Autodesk Fusion 360 part; units mm, degrees
note: some values were not read from the file. Set by a fixed rule: which sketch regions a step uses.
(part 3 of 15)
  line L1668 (302.273, -82.2438) -> (302.188, -82.0789)
  line L1669 (24.5588, -81.825) -> (24.4325, -81.5723)
  line L1670 (32.1614, -81.3271) -> (32.215, -81.5045)
  line L1671 (302.388, -82.3891) -> (302.273, -82.2438)
  line L1672 (302.137, -81.9006) -> (302.122, -81.7159)
  line L1673 (302.198, -81.3549) -> (302.288, -81.1924)
  line L1674 (303.95, -81.3671) -> (304.003, -81.5446)
  line L1675 (303.052, -82.6789) -> (302.867, -82.657)
  line L1676 (303.236, -82.6647) -> (303.052, -82.6789)
  line L1677 (32.0744, -81.1633) -> (32.1614, -81.3271)
  line L1678 (31.4741, -80.7585) -> (31.6512, -80.8133)
  line L1679 (302.188, -82.0789) -> (302.137, -81.9006)
  line L1680 (302.142, -81.5316) -> (302.198, -81.3549)
  line L1681 (302.407, -81.0504) -> (302.551, -80.9342)
  line L1682 (302.716, -80.8483) -> (302.893, -80.796)
  line L1683 (31.6512, -80.8133) -> (31.8143, -80.9015)
  line L1684 (31.8143, -80.9015) -> (31.9572, -81.0197)
  line L1685 (24.801, -79.4609) -> (25.0054, -79.2659)
  line L1686 (25.2353, -79.1017) -> (25.486, -78.9714)
  line L1687 (303.746, -81.0597) -> (303.863, -81.2034)
  line L1688 (24.2812, -80.7441) -> (24.31, -80.4631)
  line L1689 (304.003, -81.5446) -> (304.021, -81.7291)
  line L1690 (303.262, -80.7985) -> (303.44, -80.8534)
  line L1691 (85.9153, -105.918) -> (85.7941, -106.059)
  line L1692 (84.7587, -106.241) -> (84.5968, -106.151)
  line L1693 (274.699, -101.972) -> (274.897, -102.173)
  line L1694 (84.5968, -106.151) -> (84.4556, -106.031)
  line L1695 (-66.507, -105.451) -> (-66.5655, -105.627)
  line L1696 (-68.3832, -105.227) -> (-68.3626, -105.043)
  line L1697 (274.897, -102.173) -> (275.065, -102.4)
  line L1698 (85.1191, -106.321) -> (84.935, -106.299)
  line L1699 (84.3404, -105.885) -> (84.2557, -105.721)
  line L1700 (84.2097, -105.173) -> (84.2658, -104.997)
  line L1701 (-66.7782, -105.929) -> (-66.9243, -106.043)
  line L1702 (-67.2684, -106.176) -> (-67.4532, -106.19)
  line L1703 (84.1891, -105.358) -> (84.2097, -105.173)
  line L1704 (-66.9243, -106.043) -> (-67.0898, -106.126)
  line L1705 (85.1456, -104.421) -> (85.33, -104.44)
  line L1706 (84.2658, -104.997) -> (84.3551, -104.834)
  line L1707 (-67.0652, -104.365) -> (-66.9021, -104.453)
  line L1708 (-67.4532, -106.19) -> (-67.6373, -106.168)
  line L1709 (-68.3677, -105.412) -> (-68.3832, -105.227)
  line L1710 (-67.4267, -104.291) -> (-67.2423, -104.31)
  line L1711 (-68.098, -104.562) -> (-67.9535, -104.446)
  line L1712 (273.689, -101.497) -> (273.964, -101.56)
  line L1713 (84.935, -106.299) -> (84.7587, -106.241)
  line L1714 (84.4556, -106.031) -> (84.3404, -105.885)
  line L1715 (274.474, -101.8) -> (274.699, -101.972)
  line L1716 (-68.3166, -105.59) -> (-68.3677, -105.412)
  line L1717 (273.964, -101.56) -> (274.227, -101.662)
  line L1718 (-68.3626, -105.043) -> (-68.3065, -104.866)
  line L1719 (-67.6114, -104.307) -> (-67.4267, -104.291)
  line L1720 (-68.3065, -104.866) -> (-68.2172, -104.704)
  line L1721 (274.227, -101.662) -> (274.474, -101.8)
  line L1722 (275.065, -102.4) -> (275.199, -102.649)
  line L1723 (86.0173, -105.009) -> (86.0709, -105.186)
  line L1724 (249.992, -105.959) -> (249.871, -106.099)
  line L1725 (78.199, -104.986) -> (78.1482, -104.708)
  line L1726 (78.4147, -105.507) -> (78.2884, -105.254)
  line L1727 (85.9303, -104.845) -> (86.0173, -105.009)
  line L1728 (248.432, -104.874) -> (248.551, -104.732)
  line L1729 (86.089, -105.371) -> (86.0886, -105.397)
  line L1730 (249.38, -106.346) -> (249.196, -106.361)
  line L1731 (78.6569, -103.143) -> (78.8613, -102.948)
  line L1732 (248.551, -104.732) -> (248.695, -104.616)
  line L1733 (78.2884, -105.254) -> (78.199, -104.986)
  line L1734 (250.166, -105.411) -> (250.165, -105.437)
  line L1735 (250.165, -105.437) -> (250.142, -105.621)
  line L1736 (79.2282, -106.271) -> (78.9861, -106.125)
  line L1737 (78.234, -103.871) -> (78.3401, -103.609)
  line L1738 (250.007, -104.885) -> (250.094, -105.049)
  line L1739 (248.532, -106.071) -> (248.417, -105.926)
  line L1740 (249.012, -106.339) -> (248.835, -106.281)
  line L1741 (85.6702, -104.583) -> (85.8131, -104.701)
  line L1742 (248.286, -105.213) -> (248.342, -105.037)
  line L1743 (86.0709, -105.186) -> (86.089, -105.371)
  line L1744 (86.0886, -105.397) -> (86.0654, -105.581)
  line L1745 (249.559, -106.297) -> (249.38, -106.346)
  line L1746 (85.5071, -104.495) -> (85.6702, -104.583)
  line L1747 (250.147, -105.226) -> (250.166, -105.411)
  line L1748 (78.8613, -102.948) -> (79.0912, -102.783)
  line L1749 (78.1482, -104.708) -> (78.1371, -104.426)
  line L1750 (79.0912, -102.783) -> (79.3419, -102.653)
  line L1751 (78.1371, -104.426) -> (78.1659, -104.145)
  line L1752 (249.196, -106.361) -> (249.012, -106.339)
  line L1753 (85.33, -104.44) -> (85.5071, -104.495)
  line L1754 (248.332, -105.761) -> (248.281, -105.582)
  line L1755 (250.142, -105.621) -> (250.083, -105.797)
  line L1756 (249.222, -104.461) -> (249.407, -104.48)
  line L1757 (248.673, -106.191) -> (248.532, -106.071)
  line L1758 (249.725, -106.213) -> (249.559, -106.297)
  line L1759 (85.8131, -104.701) -> (85.9303, -104.845)
  line L1760 (249.871, -106.099) -> (249.725, -106.213)
  line L1761 (248.835, -106.281) -> (248.673, -106.191)
  line L1762 (248.342, -105.037) -> (248.432, -104.874)
  line L1763 (86.0069, -105.757) -> (85.9153, -105.918)
  line L1764 (248.417, -105.926) -> (248.332, -105.761)
  line L1765 (248.266, -105.398) -> (248.286, -105.213)
  line L1766 (248.281, -105.582) -> (248.266, -105.398)
  line L1767 (250.083, -105.797) -> (249.992, -105.959)
  line L1768 (248.695, -104.616) -> (248.86, -104.53)
  line L1769 (248.86, -104.53) -> (249.038, -104.478)
  line L1770 (249.038, -104.478) -> (249.222, -104.461)
  line L1771 (84.961, -104.438) -> (85.1456, -104.421)
  line L1772 (-67.2423, -104.31) -> (-67.0652, -104.365)
  line L1773 (84.2046, -105.542) -> (84.1891, -105.358)
  line L1774 (84.6188, -104.576) -> (84.7831, -104.49)
  line L1775 (85.304, -106.306) -> (85.1191, -106.321)
  line L1776 (85.7941, -106.059) -> (85.648, -106.173)
  line L1777 (84.7831, -104.49) -> (84.961, -104.438)
  line L1778 (84.4743, -104.692) -> (84.6188, -104.576)
  line L1779 (84.3551, -104.834) -> (84.4743, -104.692)
  line L1780 (-66.7592, -104.571) -> (-66.6421, -104.715)
  line L1781 (-66.6421, -104.715) -> (-66.555, -104.879)
  line L1782 (-66.555, -104.879) -> (-66.5014, -105.056)
  line L1783 (86.0654, -105.581) -> (86.0069, -105.757)
  line L1784 (-66.9021, -104.453) -> (-66.7592, -104.571)
  line L1785 (84.2557, -105.721) -> (84.2046, -105.542)
  line L1786 (-66.4833, -105.241) -> (-66.4837, -105.267)
  line L1787 (-66.5014, -105.056) -> (-66.4833, -105.241)
  line L1788 (85.4825, -106.257) -> (85.304, -106.306)
  line L1789 (85.648, -106.173) -> (85.4825, -106.257)
  line L1790 (227.735, -91.279) -> (227.912, -91.3338)
  line L1791 (100.763, -89.5821) -> (101.013, -89.4519)
  line L1792 (228.494, -92.2361) -> (228.47, -92.42)
  line L1793 (228.412, -92.596) -> (228.32, -92.7572)
  line L1794 (100.086, -92.3055) -> (99.96, -92.0527)
  line L1795 (228.32, -92.7572) -> (228.199, -92.8975)
  line L1796 (228.335, -91.6839) -> (228.422, -91.8476)
  line L1797 (228.053, -93.0117) -> (227.887, -93.0953)
  line L1798 (227.887, -93.0953) -> (227.709, -93.1451)
  line L1799 (107.466, -92.8575) -> (107.32, -92.9716)
  line L1800 (107.342, -91.3819) -> (107.485, -91.5001)
  line L1801 (226.745, -92.7242) -> (226.661, -92.5593)
  line L1802 (227.912, -91.3338) -> (228.075, -91.422)
  line L1803 (101.557, -89.3031) -> (101.839, -89.2876)
  line L1804 (226.671, -91.8353) -> (226.76, -91.6729)
  line L1805 (107.678, -92.5559) -> (107.587, -92.7171)
  line L1806 (107.32, -92.9716) -> (107.154, -93.0552)
  line L1807 (107.179, -91.2937) -> (107.342, -91.3819)
  line L1808 (227.34, -93.1374) -> (227.164, -93.0801)
  line L1809 (227.164, -93.0801) -> (227.002, -92.9897)
  line L1810 (226.594, -92.1963) -> (226.615, -92.0121)
  line L1811 (226.615, -92.0121) -> (226.671, -91.8353)
  line L1812 (107.485, -91.5001) -> (107.602, -91.6438)
  line L1813 (107.154, -93.0552) -> (106.976, -93.1051)
  line L1814 (227.551, -91.2596) -> (227.735, -91.279)
  line L1815 (107.602, -91.6438) -> (107.689, -91.8075)
  line L1816 (227.524, -93.1594) -> (227.34, -93.1374)
  line L1817 (226.61, -92.3811) -> (226.594, -92.1963)
  line L1818 (107.743, -91.985) -> (107.761, -92.1695)
  line L1819 (226.861, -92.8695) -> (226.745, -92.7242)
  line L1820 (107.689, -91.8075) -> (107.743, -91.985)
  line L1821 (227.366, -91.2764) -> (227.551, -91.2596)
  line L1822 (107.587, -92.7171) -> (107.466, -92.8575)
  line L1823 (226.76, -91.6729) -> (226.879, -91.5308)
  line L1824 (227.188, -91.3287) -> (227.366, -91.2764)
  line L1825 (226.661, -92.5593) -> (226.61, -92.3811)
  line L1826 (107.002, -91.2389) -> (107.179, -91.2937)
  line L1827 (-17.1187, -94.0653) -> (-16.9544, -93.9794)
  line L1828 (-26.4131, -92.1654) -> (-26.236, -92.2202)
  line L1829 (-25.8129, -92.5702) -> (-25.7258, -92.7339)
  line L1830 (-27.5386, -93.2674) -> (-27.5541, -93.0827)
  line L1831 (-26.236, -92.2202) -> (-26.0729, -92.3084)
  line L1832 (-17.3824, -94.3235) -> (-17.2632, -94.1815)
  line L1833 (-17.4717, -94.486) -> (-17.3824, -94.3235)
  line L1834 (-25.6723, -92.9114) -> (-25.6542, -93.096)
  line L1835 (233.398, -89.5178) -> (233.645, -89.6558)
  line L1836 (-16.4336, -95.7958) -> (-16.6184, -95.81)
  line L1837 (-25.6778, -93.3064) -> (-25.7363, -93.4824)
  line L1838 (-17.3971, -95.3748) -> (-17.4818, -95.2099)
  line L1839 (-25.6545, -93.1225) -> (-25.6778, -93.3064)
  line L1840 (-16.9544, -93.9794) -> (-16.7765, -93.927)
  line L1841 (-26.7822, -92.1628) -> (-26.5975, -92.146)
  line L1842 (-27.5541, -93.0827) -> (-27.5334, -92.8984)
  line L1843 (-27.2688, -92.4172) -> (-27.1244, -92.301)
  line L1844 (-26.4392, -94.0315) -> (-26.6241, -94.0457)
  line L1845 (233.645, -89.6558) -> (233.869, -89.8272)
  line L1846 (232.86, -89.3521) -> (233.135, -89.4159)
  line L1847 (-26.8082, -94.0238) -> (-26.9845, -93.9665)
  line L1848 (-16.255, -95.7459) -> (-16.4336, -95.7958)
  line L1849 (-16.5919, -93.9102) -> (-16.4075, -93.9296)
  line L1850 (-16.6184, -95.81) -> (-16.8025, -95.7881)
  line L1851 (233.135, -89.4159) -> (233.398, -89.5178)
  line L1852 (-16.8025, -95.7881) -> (-16.9789, -95.7308)
  line L1853 (-17.5484, -94.847) -> (-17.5278, -94.6627)
  line L1854 (-25.9301, -92.4266) -> (-25.8129, -92.5702)
  line L1855 (-16.9789, -95.7308) -> (-17.1407, -95.6403)
  line L1856 (-16.7765, -93.927) -> (-16.5919, -93.9102)
  line L1857 (-25.6542, -93.096) -> (-25.6545, -93.1225)
  line L1858 (-25.7363, -93.4824) -> (-25.8279, -93.6436)
  line L1859 (233.869, -89.8272) -> (234.068, -90.0285)
  line L1860 (-27.2875, -93.7559) -> (-27.4027, -93.6106)
  line L1861 (-27.4773, -92.7217) -> (-27.388, -92.5592)
  line L1862 (-26.96, -92.2151) -> (-26.7822, -92.1628)
  line L1863 (234.068, -90.0285) -> (234.235, -90.2558)
  line L1864 (234.235, -90.2558) -> (234.37, -90.5044)
  line L1865 (234.37, -90.5044) -> (234.467, -90.7695)
  line L1866 (234.467, -90.7695) -> (234.527, -91.0456)
  line L1867 (234.527, -91.0456) -> (234.547, -91.3274)
  line L1868 (-26.0951, -93.8981) -> (-26.2606, -93.9817)
  line L1869 (-25.949, -93.7839) -> (-26.0951, -93.8981)
  line L1870 (-27.388, -92.5592) -> (-27.2688, -92.4172)
  line L1871 (-27.1463, -93.876) -> (-27.2875, -93.7559)
  line L1872 (-27.4875, -93.4457) -> (-27.5386, -93.2674)
  line L1873 (-27.1244, -92.301) -> (-26.96, -92.2151)
  line L1874 (-25.8279, -93.6436) -> (-25.949, -93.7839)
  line L1875 (231.752, -89.4919) -> (232.019, -89.3983)
  line L1876 (230.61, -91.8248) -> (230.559, -91.5469)
  line L1877 (230.893, -90.2033) -> (231.067, -89.9814)
  line L1878 (233.773, -92.9078) -> (233.538, -93.0647)
  line L1879 (231.178, -92.7854) -> (230.986, -92.5779)
  line L1880 (234.165, -92.503) -> (233.983, -92.7193)
  line L1881 (234.428, -92.0049) -> (234.314, -92.2633)
  line L1882 (-26.5975, -92.146) -> (-26.4131, -92.1654)
  line L1883 (-26.2606, -93.9817) -> (-26.4392, -94.0315)
  line L1884 (230.576, -90.9836) -> (230.645, -90.7094)
  line L1885 (-26.6241, -94.0457) -> (-26.8082, -94.0238)
  line L1886 (-26.9845, -93.9665) -> (-27.1463, -93.876)
  line L1887 (-27.5334, -92.8984) -> (-27.4773, -92.7217)
  line L1888 (234.314, -92.2633) -> (234.165, -92.503)
  line L1889 (230.699, -92.0928) -> (230.61, -91.8248)
  line L1890 (234.547, -91.3274) -> (234.543, -91.453)
  line L1891 (233.283, -93.187) -> (233.014, -93.2722)
  line L1892 (233.983, -92.7193) -> (233.773, -92.9078)
  line L1893 (231.397, -92.9637) -> (231.178, -92.7854)
  line L1894 (231.272, -89.7864) -> (231.502, -89.6222)
  line L1895 (233.538, -93.0647) -> (233.283, -93.187)
  line L1896 (231.502, -89.6222) -> (231.752, -89.4919)
  line L1897 (234.543, -91.453) -> (234.505, -91.733)
  line L1898 (-27.4027, -93.6106) -> (-27.4875, -93.4457)
  line L1899 (230.645, -90.7094) -> (230.751, -90.4476)
  line L1900 (230.825, -92.3455) -> (230.699, -92.0928)
  line L1901 (234.505, -91.733) -> (234.428, -92.0049)
  line L1902 (230.548, -91.2646) -> (230.576, -90.9836)
  line L1903 (232.172, -93.292) -> (231.899, -93.2196)
  line L1904 (230.751, -90.4476) -> (230.893, -90.2033)
  line L1905 (231.067, -89.9814) -> (231.272, -89.7864)
  line L1906 (232.453, -93.3252) -> (232.172, -93.292)
  line L1907 (230.986, -92.5779) -> (230.825, -92.3455)
  line L1908 (231.899, -93.2196) -> (231.639, -93.1095)
  line L1909 (230.559, -91.5469) -> (230.548, -91.2646)
  line L1910 (103.426, -92.4629) -> (103.244, -92.6792)
  line L1911 (233.014, -93.2722) -> (232.735, -93.3186)
  line L1912 (232.735, -93.3186) -> (232.453, -93.3252)
  line L1913 (103.804, -91.413) -> (103.766, -91.6929)
  line L1914 (101.433, -93.2519) -> (101.16, -93.1795)
  line L1915 (102.906, -89.6158) -> (103.13, -89.7872)
  line L1916 (102.659, -89.4777) -> (102.906, -89.6158)
  line L1917 (103.496, -90.2157) -> (103.631, -90.4643)
  line L1918 (103.034, -92.8677) -> (102.799, -93.0246)
  line L1919 (102.275, -93.2321) -> (101.996, -93.2785)
  line L1920 (103.631, -90.4643) -> (103.728, -90.7294)
  line L1921 (103.766, -91.6929) -> (103.69, -91.9649)
  line L1922 (100.247, -92.5379) -> (100.086, -92.3055)
  line L1923 (231.639, -93.1095) -> (231.397, -92.9637)
  line L1924 (102.799, -93.0246) -> (102.544, -93.1469)
  line L1925 (101.996, -93.2785) -> (101.714, -93.2852)
  line L1926 (232.296, -89.3432) -> (232.578, -89.3277)
  line L1927 (100.9, -93.0694) -> (100.658, -92.9237)
  line L1928 (100.658, -92.9237) -> (100.439, -92.7453)
  line L1929 (100.439, -92.7453) -> (100.247, -92.5379)
  line L1930 (103.329, -89.9885) -> (103.496, -90.2157)
  line L1931 (102.121, -89.312) -> (102.396, -89.3758)
  line L1932 (103.788, -91.0056) -> (103.808, -91.2874)
  line L1933 (103.13, -89.7872) -> (103.329, -89.9885)
  line L1934 (102.396, -89.3758) -> (102.659, -89.4777)
  line L1935 (103.808, -91.2874) -> (103.804, -91.413)
  line L1936 (101.714, -93.2852) -> (101.433, -93.2519)
  line L1937 (102.544, -93.1469) -> (102.275, -93.2321)
  line L1938 (227.709, -93.1451) -> (227.524, -93.1594)
  line L1939 (99.8706, -91.7848) -> (99.8199, -91.5068)
  line L1940 (100.154, -90.1632) -> (100.329, -89.9413)
  line L1941 (99.8088, -91.2246) -> (99.8376, -90.9435)
  line L1942 (100.329, -89.9413) -> (100.533, -89.7463)
  line L1943 (99.9057, -90.6693) -> (100.012, -90.4075)
  line L1944 (228.218, -91.5402) -> (228.335, -91.6839)
  line L1945 (100.533, -89.7463) -> (100.763, -89.5821)
  line L1946 (228.075, -91.422) -> (228.218, -91.5402)
  line L1947 (103.575, -92.2232) -> (103.426, -92.4629)
  line L1948 (228.422, -91.8476) -> (228.476, -92.0251)
  line L1949 (99.8199, -91.5068) -> (99.8088, -91.2246)
  line L1950 (228.476, -92.0251) -> (228.494, -92.2096)
  line L1951 (99.8376, -90.9435) -> (99.9057, -90.6693)
  line L1952 (228.494, -92.2096) -> (228.494, -92.2361)
  line L1953 (101.16, -93.1795) -> (100.9, -93.0694)
  line L1954 (103.728, -90.7294) -> (103.788, -91.0056)
  line L1955 (232.019, -89.3983) -> (232.296, -89.3432)
  line L1956 (103.244, -92.6792) -> (103.034, -92.8677)
  line L1957 (232.578, -89.3277) -> (232.86, -89.3521)
  line L1958 (103.69, -91.9649) -> (103.575, -92.2232)
  line L1959 (99.96, -92.0527) -> (99.8706, -91.7848)
  line L1960 (100.012, -90.4075) -> (100.154, -90.1632)
  line L1961 (101.28, -89.3583) -> (101.557, -89.3031)
  line L1962 (101.013, -89.4519) -> (101.28, -89.3583)
  line L1963 (228.199, -92.8975) -> (228.053, -93.0117)
  line L1964 (228.47, -92.42) -> (228.412, -92.596)
  line L1965 (101.839, -89.2876) -> (102.121, -89.312)
  line L1966 (288.551, -103.613) -> (288.569, -103.798)
  line L1967 (287.599, -104.748) -> (287.415, -104.726)
  line L1968 (47.614, -103.396) -> (47.6676, -103.573)
  line L1969 (287.238, -104.668) -> (287.077, -104.578)
  line L1970 (288.128, -104.6) -> (287.962, -104.683)
  line L1971 (286.935, -104.458) -> (286.82, -104.312)
  line L1972 (287.784, -104.733) -> (287.599, -104.748)
  line L1973 (287.263, -102.917) -> (287.441, -102.865)
  line L1974 (287.077, -104.578) -> (286.935, -104.458)
  line L1975 (47.3908, -104.446) -> (47.2447, -104.56)
  line L1976 (39.7957, -103.373) -> (39.7449, -103.095)
  line L1977 (40.2536, -101.529) -> (40.458, -101.334)
  line L1978 (288.569, -103.798) -> (288.568, -103.824)
  line L1979 (286.736, -104.147) -> (286.684, -103.969)
  line L1980 (40.458, -101.334) -> (40.6879, -101.17)
  line L1981 (286.669, -103.784) -> (286.69, -103.6)
  line L1982 (288.395, -104.345) -> (288.274, -104.486)
  line L1983 (41.7643, -100.876) -> (42.0457, -100.9)
  line L1984 (287.987, -102.922) -> (288.15, -103.01)
  line L1985 (288.274, -104.486) -> (288.128, -104.6)
  line L1986 (288.568, -103.824) -> (288.545, -104.008)
  line L1987 (40.6879, -101.17) -> (40.9386, -101.04)
  line L1988 (287.962, -104.683) -> (287.784, -104.733)
  line L1989 (288.41, -103.272) -> (288.497, -103.436)
  line L1990 (39.7626, -102.532) -> (39.8307, -102.257)
  line L1991 (47.2669, -102.97) -> (47.4098, -103.088)
  line L1992 (47.2447, -104.56) -> (47.0792, -104.643)
  line L1993 (288.545, -104.008) -> (288.487, -104.184)
  line L1994 (47.512, -104.305) -> (47.3908, -104.446)
  line L1995 (41.4822, -100.891) -> (41.7643, -100.876)
  line L1996 (286.684, -103.969) -> (286.669, -103.784)
  line L1997 (287.415, -104.726) -> (287.238, -104.668)
  line L1998 (46.9267, -102.827) -> (47.1038, -102.882)
  line L1999 (47.527, -103.232) -> (47.614, -103.396)
  line L2000 (47.6621, -103.968) -> (47.6035, -104.144)
  line L2001 (46.9006, -104.693) -> (46.7158, -104.707)
  line L2002 (47.6035, -104.144) -> (47.512, -104.305)
  line L2003 (286.746, -103.423) -> (286.835, -103.261)
  line L2004 (47.0792, -104.643) -> (46.9006, -104.693)
  line L2005 (287.099, -103.003) -> (287.263, -102.917)
  line L2006 (287.625, -102.848) -> (287.81, -102.867)
  line L2007 (286.82, -104.312) -> (286.736, -104.147)
  line L2008 (286.835, -103.261) -> (286.954, -103.119)
  line L2009 (286.69, -103.6) -> (286.746, -103.423)
  line L2010 (260.153, -103.462) -> (260.171, -103.647)
  line L2011 (47.1038, -102.882) -> (47.2669, -102.97)
  line L2012 (46.5577, -102.824) -> (46.7423, -102.808)
  line L2013 (260.099, -103.285) -> (260.153, -103.462)
  line L2014 (259.997, -104.194) -> (259.876, -104.335)
  line L2015 (47.6857, -103.758) -> (47.6853, -103.784)
  line L2016 (286.954, -103.119) -> (287.099, -103.003)
  line L2017 (287.441, -102.865) -> (287.625, -102.848)
  line L2018 (260.089, -104.033) -> (259.997, -104.194)
  line L2019 (259.876, -104.335) -> (259.73, -104.449)
  line L2020 (45.9371, -104.272) -> (45.8524, -104.107)
  line L2021 (47.6853, -103.784) -> (47.6621, -103.968)
  line L2022 (260.148, -103.857) -> (260.089, -104.033)
  line L2023 (47.4098, -103.088) -> (47.527, -103.232)
  line L2024 (45.7858, -103.744) -> (45.8064, -103.56)
  line L2025 (259.565, -104.532) -> (259.386, -104.582)
  line L2026 (46.3798, -102.877) -> (46.5577, -102.824)
  line L2027 (46.5317, -104.685) -> (46.3553, -104.628)
  line L2028 (47.6676, -103.573) -> (47.6857, -103.758)
  line L2029 (46.0523, -104.418) -> (45.9371, -104.272)
  line L2030 (46.2155, -102.963) -> (46.3798, -102.877)
  line L2031 (259.73, -104.449) -> (259.565, -104.532)
  line L2032 (46.1935, -104.538) -> (46.0523, -104.418)
  line L2033 (46.071, -103.079) -> (46.2155, -102.963)
  line L2034 (45.8013, -103.929) -> (45.7858, -103.744)
  line L2035 (45.9518, -103.221) -> (46.071, -103.079)
  line L2036 (45.8625, -103.383) -> (45.9518, -103.221)
  line L2037 (46.7423, -102.808) -> (46.9267, -102.827)
  line L2038 (259.589, -102.771) -> (259.752, -102.859)
  line L2039 (46.3553, -104.628) -> (46.1935, -104.538)
  line L2040 (259.412, -102.716) -> (259.589, -102.771)
  line L2041 (260.012, -103.121) -> (260.099, -103.285)
  line L2042 (260.171, -103.647) -> (260.171, -103.673)
  line L2043 (260.171, -103.673) -> (260.148, -103.857)
  line L2044 (259.752, -102.859) -> (259.895, -102.977)
  line L2045 (45.8524, -104.107) -> (45.8013, -103.929)
  line L2046 (45.8064, -103.56) -> (45.8625, -103.383)
  line L2047 (46.7158, -104.707) -> (46.5317, -104.685)
  line L2048 (258.338, -103.996) -> (258.287, -103.818)
  line L2049 (74.6132, -102.812) -> (74.7775, -102.726)
  line L2050 (259.017, -104.574) -> (258.841, -104.517)
  line L2051 (259.201, -104.596) -> (259.017, -104.574)
  line L2052 (258.348, -103.272) -> (258.437, -103.11)
  line L2053 (76.0117, -103.245) -> (76.0652, -103.422)
  line L2054 (258.701, -102.852) -> (258.865, -102.766)
  line L2055 (259.386, -104.582) -> (259.201, -104.596)
  line L2056 (75.9096, -104.154) -> (75.7885, -104.295)
  line L2057 (75.7885, -104.295) -> (75.6424, -104.409)
  line L2058 (258.679, -104.427) -> (258.538, -104.307)
  line L2059 (76.0833, -103.607) -> (76.083, -103.633)
  line L2060 (258.423, -104.161) -> (258.338, -103.996)
  line L2061 (75.5015, -102.731) -> (75.6646, -102.819)
  line L2062 (258.841, -104.517) -> (258.679, -104.427)
  line L2063 (76.0597, -103.817) -> (76.0012, -103.993)
  line L2064 (258.287, -103.818) -> (258.271, -103.633)
  line L2065 (258.538, -104.307) -> (258.423, -104.161)
  line L2066 (76.0652, -103.422) -> (76.0833, -103.607)
  line L2067 (76.083, -103.633) -> (76.0597, -103.817)
  line L2068 (258.271, -103.633) -> (258.292, -103.449)
  line L2069 (75.6424, -104.409) -> (75.4769, -104.492)
  line L2070 (75.14, -102.657) -> (75.3244, -102.676)
  line L2071 (278.91, -101.802) -> (279.053, -101.92)
  line L2072 (74.5912, -104.387) -> (74.45, -104.266)
  line L2073 (258.292, -103.449) -> (258.348, -103.272)
  line L2074 (76.0012, -103.993) -> (75.9096, -104.154)
  line L2075 (258.437, -103.11) -> (258.556, -102.968)
  line L2076 (259.043, -102.713) -> (259.228, -102.697)
  line L2077 (258.865, -102.766) -> (259.043, -102.713)
  line L2078 (74.3348, -104.121) -> (74.2501, -103.956)
  line L2079 (75.9246, -103.081) -> (76.0117, -103.245)
  line L2080 (75.2983, -104.542) -> (75.1134, -104.556)
  line L2081 (259.228, -102.697) -> (259.412, -102.716)
  line L2082 (75.3244, -102.676) -> (75.5015, -102.731)
  line L2083 (74.7775, -102.726) -> (74.9553, -102.673)
  line L2084 (258.556, -102.968) -> (258.701, -102.852)
  line L2085 (75.8074, -102.937) -> (75.9246, -103.081)
  line L2086 (259.895, -102.977) -> (260.012, -103.121)
  line L2087 (75.6646, -102.819) -> (75.8074, -102.937)
  line L2088 (74.9553, -102.673) -> (75.14, -102.657)
  line L2089 (75.1134, -104.556) -> (74.9293, -104.534)
  line L2090 (74.1834, -103.593) -> (74.2041, -103.409)
  line L2091 (279.311, -102.405) -> (279.329, -102.59)
  line L2092 (279.17, -102.064) -> (279.257, -102.228)
  line L2093 (295.167, -141.134) -> (295.185, -141.319)
  line L2094 (295.185, -141.319) -> (295.184, -141.345)
  line L2095 (294.578, -142.205) -> (294.4, -142.254)
  line L2096 (293.57, -140.64) -> (293.715, -140.524)
  line L2097 (293.352, -141.669) -> (293.3, -141.49)
  line L2098 (294.031, -142.247) -> (293.854, -142.189)
  line L2099 (39.2364, -141.629) -> (39.1853, -141.45)
  line L2100 (39.1853, -141.45) -> (39.1698, -141.266)
  line L2101 (40.896, -141.826) -> (40.7748, -141.967)
  line L2102 (40.2846, -142.214) -> (40.0998, -142.229)
  line L2103 (294.241, -140.369) -> (294.426, -140.388)
  line L2104 (293.879, -140.438) -> (294.057, -140.386)
  line L2105 (39.4363, -141.939) -> (39.3211, -141.793)
  line L2106 (293.436, -141.834) -> (293.352, -141.669)
  line L2107 (293.285, -141.306) -> (293.306, -141.121)
  line L2108 (40.7748, -141.967) -> (40.6287, -142.081)
  line L2109 (40.0998, -142.229) -> (39.9157, -142.207)
  line L2110 (39.7393, -142.149) -> (39.5775, -142.059)
  line L2111 (295.103, -141.705) -> (295.011, -141.867)
  line L2112 (40.4878, -140.403) -> (40.6509, -140.491)
  line L2113 (40.7938, -140.609) -> (40.911, -140.753)
  line L2114 (41.0461, -141.489) -> (40.9875, -141.665)
  line L2115 (294.426, -140.388) -> (294.603, -140.443)
  line L2116 (294.215, -142.269) -> (294.031, -142.247)
  line L2117 (40.3107, -140.348) -> (40.4878, -140.403)
  line L2118 (39.3358, -140.742) -> (39.455, -140.6)
  line L2119 (293.306, -141.121) -> (293.362, -140.945)
  line L2120 (295.026, -140.793) -> (295.113, -140.957)
  line L2121 (294.89, -142.007) -> (294.744, -142.121)
  line L2122 (295.011, -141.867) -> (294.89, -142.007)
  line L2123 (294.744, -142.121) -> (294.578, -142.205)
  line L2124 (41.0516, -141.094) -> (41.0697, -141.279)
  line L2125 (39.3211, -141.793) -> (39.2364, -141.629)
  line L2126 (295.113, -140.957) -> (295.167, -141.134)
  line L2127 (39.1904, -141.081) -> (39.2465, -140.905)
  line L2128 (34.8662, -138.412) -> (35.1483, -138.397)
  line L2129 (294.909, -140.649) -> (295.026, -140.793)
  line L2130 (294.766, -140.531) -> (294.909, -140.649)
  line L2131 (39.2465, -140.905) -> (39.3358, -140.742)
  line L2132 (39.455, -140.6) -> (39.5995, -140.484)
  line L2133 (40.9875, -141.665) -> (40.896, -141.826)
  line L2134 (294.057, -140.386) -> (294.241, -140.369)
  line L2135 (293.854, -142.189) -> (293.693, -142.099)
  line L2136 (294.4, -142.254) -> (294.215, -142.269)
  line L2137 (39.1698, -141.266) -> (39.1904, -141.081)
  line L2138 (293.693, -142.099) -> (293.551, -141.979)
  line L2139 (295.184, -141.345) -> (295.161, -141.529)
  line L2140 (293.451, -140.782) -> (293.57, -140.64)
  line L2141 (35.1483, -138.397) -> (35.4297, -138.421)
  line L2142 (294.603, -140.443) -> (294.766, -140.531)
  line L2143 (264.887, -141.155) -> (264.908, -140.97)
  line L2144 (266.205, -140.292) -> (266.368, -140.38)
  line L2145 (68.6823, -142.063) -> (68.4974, -142.078)
  line L2146 (69.3852, -141.514) -> (69.2936, -141.675)
  line L2147 (40.1263, -140.329) -> (40.3107, -140.348)
  line L2148 (266.613, -141.715) -> (266.492, -141.856)
  line L2149 (265.154, -141.828) -> (265.039, -141.682)
  line L2150 (265.295, -141.948) -> (265.154, -141.828)
  line L2151 (265.457, -142.038) -> (265.295, -141.948)
  line L2152 (39.5995, -140.484) -> (39.7638, -140.398)
  line L2153 (266.764, -141.378) -> (266.705, -141.554)
  line L2154 (69.467, -141.154) -> (69.4437, -141.338)
  line L2155 (67.6341, -141.477) -> (67.5829, -141.299)
  line L2156 (67.5829, -141.299) -> (67.5674, -141.114)
  line L2157 (67.834, -141.788) -> (67.7188, -141.642)
  line L2158 (67.5674, -141.114) -> (67.5881, -140.93)
  line L2159 (67.9752, -141.908) -> (67.834, -141.788)
  line L2160 (69.4673, -141.128) -> (69.467, -141.154)
  line L2161 (266.511, -140.498) -> (266.628, -140.642)
  line L2162 (266.787, -141.194) -> (266.764, -141.378)
  line L2163 (69.0486, -140.34) -> (69.1914, -140.458)
  line L2164 (265.659, -140.235) -> (265.844, -140.218)
  line L2165 (69.0264, -141.93) -> (68.8609, -142.013)
  line L2166 (39.5775, -142.059) -> (39.4363, -141.939)
  line L2167 (68.8609, -142.013) -> (68.6823, -142.063)
  line L2168 (39.9157, -142.207) -> (39.7393, -142.149)
  line L2169 (68.3133, -142.056) -> (68.137, -141.998)
  line L2170 (67.5881, -140.93) -> (67.6442, -140.753)
  line L2171 (266.705, -141.554) -> (266.613, -141.715)
  line L2172 (39.7638, -140.398) -> (39.9417, -140.346)
  line L2173 (67.6442, -140.753) -> (67.7335, -140.591)
  line L2174 (68.137, -141.998) -> (67.9752, -141.908)
  line L2175 (265.481, -140.287) -> (265.659, -140.235)
  line L2176 (266.769, -140.983) -> (266.787, -141.168)
  line L2177 (69.2936, -141.675) -> (69.1725, -141.816)
  line L2178 (69.1914, -140.458) -> (69.3086, -140.602)
  line L2179 (265.633, -142.096) -> (265.457, -142.038)
  line L2180 (265.039, -141.682) -> (264.954, -141.518)
  line L2181 (266.028, -140.237) -> (266.205, -140.292)
  line L2182 (266.715, -140.806) -> (266.769, -140.983)
  line L2183 (266.368, -140.38) -> (266.511, -140.498)
  line L2184 (40.998, -140.917) -> (41.0516, -141.094)
  line L2185 (264.954, -141.518) -> (264.903, -141.339)
  line L2186 (266.181, -142.054) -> (266.002, -142.103)
  line L2187 (69.1725, -141.816) -> (69.0264, -141.93)
  line L2188 (265.817, -142.118) -> (265.633, -142.096)
  line L2189 (264.903, -141.339) -> (264.887, -141.155)
  line L2190 (69.3086, -140.602) -> (69.3957, -140.766)
  line L2191 (40.6509, -140.491) -> (40.7938, -140.609)
  line L2192 (41.0693, -141.305) -> (41.0461, -141.489)
  line L2193 (264.964, -140.794) -> (265.053, -140.631)
  line L2194 (266.002, -142.103) -> (265.817, -142.118)
  line L2195 (40.911, -140.753) -> (40.998, -140.917)
  line L2196 (266.787, -141.168) -> (266.787, -141.194)
  line L2197 (39.9417, -140.346) -> (40.1263, -140.329)
  line L2198 (266.492, -141.856) -> (266.346, -141.97)
  line L2199 (67.7188, -141.642) -> (67.6341, -141.477)
  line L2200 (40.4632, -142.165) -> (40.2846, -142.214)
  line L2201 (265.053, -140.631) -> (265.172, -140.489)
  line L2202 (266.628, -140.642) -> (266.715, -140.806)
  line L2203 (41.0697, -141.279) -> (41.0693, -141.305)
  line L2204 (264.908, -140.97) -> (264.964, -140.794)
  line L2205 (40.6287, -142.081) -> (40.4632, -142.165)
  line L2206 (266.346, -141.97) -> (266.181, -142.054)
  line L2207 (284.614, -140.982) -> (284.453, -140.891)
  line L2208 (69.4492, -140.943) -> (69.4673, -141.128)
  line L2209 (284.111, -140.461) -> (284.06, -140.283)
  line L2210 (284.196, -140.626) -> (284.111, -140.461)
  line L2211 (284.975, -141.061) -> (284.791, -141.039)
  line L2212 (69.4437, -141.338) -> (69.3852, -141.514)
  line L2213 (284.065, -139.914) -> (284.122, -139.737)
  line L2214 (284.453, -140.891) -> (284.311, -140.771)
  line L2215 (67.9972, -140.333) -> (68.1615, -140.247)
  line L2216 (285.873, -139.749) -> (285.927, -139.927)
  line L2217 (68.524, -140.178) -> (68.7084, -140.197)
  line L2218 (285.786, -139.585) -> (285.873, -139.749)
  line L2219 (68.8855, -140.252) -> (69.0486, -140.34)
  line L2220 (265.172, -140.489) -> (265.317, -140.373)
  line L2221 (284.06, -140.283) -> (284.045, -140.098)
  line L2222 (67.7335, -140.591) -> (67.8527, -140.449)
  line L2223 (284.791, -141.039) -> (284.614, -140.982)
  line L2224 (285.186, -139.18) -> (285.363, -139.235)
  line L2225 (48.8176, -140.851) -> (48.6764, -140.731)
  line L2226 (285.921, -140.322) -> (285.863, -140.497)
  line L2227 (284.311, -140.771) -> (284.196, -140.626)
  line L2228 (265.317, -140.373) -> (265.481, -140.287)
  line L2229 (285.504, -140.913) -> (285.338, -140.997)
  line L2230 (285.927, -139.927) -> (285.945, -140.111)
  line L2231 (50.1361, -140.619) -> (50.0149, -140.759)
  line L2232 (285.669, -139.442) -> (285.786, -139.585)
  line L2233 (285.863, -140.497) -> (285.771, -140.659)
  line L2234 (67.8527, -140.449) -> (67.9972, -140.333)
  line L2235 (68.4974, -142.078) -> (68.3133, -142.056)
  line L2236 (285.65, -140.799) -> (285.504, -140.913)
  line L2237 (285.526, -139.323) -> (285.669, -139.442)
  line L2238 (285.944, -140.138) -> (285.921, -140.322)
  line L2239 (68.7084, -140.197) -> (68.8855, -140.252)
  line L2240 (50.1511, -139.545) -> (50.2381, -139.709)
  line L2241 (285.771, -140.659) -> (285.65, -140.799)
  line L2242 (68.1615, -140.247) -> (68.3393, -140.195)
  line L2243 (285.363, -139.235) -> (285.526, -139.323)
  line L2244 (285.945, -140.111) -> (285.944, -140.138)
  line L2245 (285.16, -141.047) -> (284.975, -141.061)
  line L2246 (285.338, -140.997) -> (285.16, -141.047)
  line L2247 (284.211, -139.574) -> (284.33, -139.432)
  line L2248 (50.2917, -139.886) -> (50.3098, -140.071)
  line L2249 (69.3957, -140.766) -> (69.4492, -140.943)
  line L2250 (284.045, -140.098) -> (284.065, -139.914)
  line L2251 (68.3393, -140.195) -> (68.524, -140.178)
  line L2252 (49.1558, -140.999) -> (48.9795, -140.942)
  line L2253 (265.844, -140.218) -> (266.028, -140.237)
  line L2254 (284.122, -139.737) -> (284.211, -139.574)
  line L2255 (48.6764, -140.731) -> (48.5613, -140.586)
  line L2256 (49.5248, -141.007) -> (49.3399, -141.021)
  line L2257 (48.4254, -140.243) -> (48.4099, -140.058)
  line L2258 (49.8688, -140.873) -> (49.7033, -140.957)
  line L2259 (48.9795, -140.942) -> (48.8176, -140.851)
  line L2260 (284.639, -139.23) -> (284.817, -139.178)
  line L2261 (50.2862, -140.281) -> (50.2277, -140.457)
  line L2262 (285.001, -139.161) -> (285.186, -139.18)
  line L2263 (48.6951, -139.392) -> (48.8396, -139.276)
  line L2264 (304.609, -138.679) -> (304.772, -138.767)
  line L2265 (48.5759, -139.534) -> (48.6951, -139.392)
  line L2266 (48.4866, -139.697) -> (48.5759, -139.534)
  line L2267 (48.4099, -140.058) -> (48.4306, -139.873)
  line L2268 (304.772, -138.767) -> (304.915, -138.885)
  line L2269 (49.3664, -139.121) -> (49.5508, -139.14)
  line L2270 (303.442, -140.069) -> (303.357, -139.904)
  line L2271 (305.172, -139.37) -> (305.19, -139.555)
  line L2272 (49.5508, -139.14) -> (49.7279, -139.195)
  line L2273 (304.036, -140.482) -> (303.86, -140.425)
  line L2274 (303.698, -140.335) -> (303.557, -140.215)
  line L2275 (303.557, -140.215) -> (303.442, -140.069)
  line L2276 (304.221, -140.504) -> (304.036, -140.482)
  line L2277 (49.891, -139.283) -> (50.0339, -139.402)
  line L2278 (305.032, -139.029) -> (305.119, -139.193)
  line L2279 (48.5613, -140.586) -> (48.4765, -140.421)
  line L2280 (50.2381, -139.709) -> (50.2917, -139.886)
  line L2281 (50.0339, -139.402) -> (50.1511, -139.545)
  line L2282 (50.0149, -140.759) -> (49.8688, -140.873)
  line L2283 (284.33, -139.432) -> (284.475, -139.316)
  line L2284 (48.4765, -140.421) -> (48.4254, -140.243)
  line L2285 (50.3094, -140.098) -> (50.2862, -140.281)
  line L2286 (284.475, -139.316) -> (284.639, -139.23)
  line L2287 (49.1818, -139.138) -> (49.3664, -139.121)
  line L2288 (304.431, -138.624) -> (304.609, -138.679)
  line L2289 (305.119, -139.193) -> (305.172, -139.37)
  line L2290 (284.817, -139.178) -> (285.001, -139.161)
  line L2291 (49.7279, -139.195) -> (49.891, -139.283)
  line L2292 (50.3098, -140.071) -> (50.3094, -140.098)
  line L2293 (50.2277, -140.457) -> (50.1361, -140.619)
  line L2294 (49.7033, -140.957) -> (49.5248, -141.007)
  line L2295 (49.3399, -141.021) -> (49.1558, -140.999)
  line L2296 (304.584, -140.44) -> (304.405, -140.49)
  line L2297 (304.405, -140.49) -> (304.221, -140.504)
  line L2298 (49.0039, -139.19) -> (49.1818, -139.138)
  line L2299 (48.4306, -139.873) -> (48.4866, -139.697)
  line L2300 (305.167, -139.765) -> (305.108, -139.941)
  line L2301 (304.896, -140.243) -> (304.75, -140.357)
  line L2302 (305.19, -139.555) -> (305.19, -139.581)
  line L2303 (304.915, -138.885) -> (305.032, -139.029)
  line L2304 (305.017, -140.102) -> (304.896, -140.243)
  line L2305 (305.19, -139.581) -> (305.167, -139.765)
  line L2306 (48.8396, -139.276) -> (49.0039, -139.19)
  line L2307 (304.75, -140.357) -> (304.584, -140.44)
  line L2308 (31.0404, -139.725) -> (30.9819, -139.901)
  line L2309 (303.367, -139.18) -> (303.457, -139.018)
  line L2310 (30.6231, -140.317) -> (30.4576, -140.4)
  line L2311 (303.576, -138.876) -> (303.72, -138.76)
  line L2312 (303.457, -139.018) -> (303.576, -138.876)
  line L2313 (303.306, -139.726) -> (303.291, -139.541)
  line L2314 (303.885, -138.674) -> (304.062, -138.621)
  line L2315 (304.247, -138.605) -> (304.431, -138.624)
  line L2316 (303.86, -140.425) -> (303.698, -140.335)
  line L2317 (303.291, -139.541) -> (303.311, -139.357)
  line L2318 (305.108, -139.941) -> (305.017, -140.102)
  line L2319 (304.062, -138.621) -> (304.247, -138.605)
  line L2320 (303.357, -139.904) -> (303.306, -139.726)
  line L2321 (29.4307, -140.174) -> (29.3155, -140.029)
  line L2322 (30.0941, -140.464) -> (29.91, -140.442)
  line L2323 (31.0637, -139.541) -> (31.0404, -139.725)
  line L2324 (30.9819, -139.901) -> (30.8903, -140.062)
  line L2325 (303.72, -138.76) -> (303.885, -138.674)
  line L2326 (303.311, -139.357) -> (303.367, -139.18)
  line L2327 (30.9924, -139.153) -> (31.0459, -139.33)
  line L2328 (29.7337, -140.385) -> (29.5719, -140.295)
  line L2329 (29.2307, -139.864) -> (29.1796, -139.686)
  line L2330 (31.064, -139.515) -> (31.0637, -139.541)
  line L2331 (30.9053, -138.989) -> (30.9924, -139.153)
  line L2332 (29.5719, -140.295) -> (29.4307, -140.174)
  line L2333 (29.3155, -140.029) -> (29.2307, -139.864)
  line L2334 (30.4576, -140.4) -> (30.279, -140.45)
  line L2335 (30.4822, -138.639) -> (30.6453, -138.727)
  line L2336 (30.6453, -138.727) -> (30.7881, -138.845)
  line L2337 (30.7692, -140.203) -> (30.6231, -140.317)
  line L2338 (30.3051, -138.584) -> (30.4822, -138.639)
  line L2339 (204.035, -137.841) -> (203.997, -138.121)
  line L2340 (29.7582, -138.634) -> (29.936, -138.581)
  line L2341 (203.029, -139.453) -> (202.775, -139.575)
  line L2342 (202.505, -139.661) -> (202.227, -139.707)
  line L2343 (29.1848, -139.317) -> (29.2409, -139.14)
  line L2344 (203.137, -136.044) -> (203.361, -136.216)
  line L2345 (29.936, -138.581) -> (30.1207, -138.565)
  line L2346 (204.019, -137.434) -> (204.038, -137.716)
  line L2347 (202.89, -135.906) -> (203.137, -136.044)
  line L2348 (203.861, -136.893) -> (203.959, -137.158)
  line L2349 (203.657, -138.891) -> (203.475, -139.108)
  line L2350 (203.806, -138.652) -> (203.657, -138.891)
  line L2351 (30.7881, -138.845) -> (30.9053, -138.989)
  line L2352 (31.0459, -139.33) -> (31.064, -139.515)
  line L2353 (30.8903, -140.062) -> (30.7692, -140.203)
  line L2354 (30.279, -140.45) -> (30.0941, -140.464)
  line L2355 (29.91, -140.442) -> (29.7337, -140.385)
  line L2356 (202.227, -139.707) -> (201.944, -139.714)
  line L2357 (203.959, -137.158) -> (204.019, -137.434)
  line L2358 (29.4494, -138.836) -> (29.5938, -138.72)
  line L2359 (202.775, -139.575) -> (202.505, -139.661)
  line L2360 (29.3302, -138.978) -> (29.4494, -138.836)
  line L2361 (203.997, -138.121) -> (203.92, -138.393)
  line L2362 (29.1796, -139.686) -> (29.1641, -139.501)
  line L2363 (202.351, -135.741) -> (202.627, -135.804)
  line L2364 (202.627, -135.804) -> (202.89, -135.906)
  line L2365 (203.92, -138.393) -> (203.806, -138.652)
  line L2366 (201.664, -139.68) -> (201.391, -139.608)
  line L2367 (200.068, -137.372) -> (200.136, -137.098)
  line L2368 (29.2409, -139.14) -> (29.3302, -138.978)
  line L2369 (29.1641, -139.501) -> (29.1848, -139.317)
  line L2370 (203.475, -139.108) -> (203.264, -139.296)
  line L2371 (30.1207, -138.565) -> (30.3051, -138.584)
  line L2372 (200.669, -139.174) -> (200.478, -138.966)
  line L2373 (200.384, -136.592) -> (200.559, -136.37)
  line L2374 (201.944, -139.714) -> (201.664, -139.68)
  line L2375 (203.361, -136.216) -> (203.559, -136.417)
  line L2376 (200.039, -137.653) -> (200.068, -137.372)
  line L2377 (203.264, -139.296) -> (203.029, -139.453)
  line L2378 (200.888, -139.352) -> (200.669, -139.174)
  line L2379 (29.5938, -138.72) -> (29.7582, -138.634)
  line L2380 (203.559, -136.417) -> (203.727, -136.644)
  line L2381 (203.727, -136.644) -> (203.861, -136.893)
  line L2382 (204.038, -137.716) -> (204.035, -137.841)
  line L2383 (201.511, -135.787) -> (201.788, -135.732)
  line L2384 (132.904, -135.764) -> (133.168, -135.866)
  line L2385 (200.317, -138.734) -> (200.191, -138.481)
  line L2386 (130.837, -136.33) -> (131.041, -136.135)
  line L2387 (130.414, -137.058) -> (130.52, -136.796)
  line L2388 (202.07, -135.716) -> (202.351, -135.741)
  line L2389 (134.084, -138.612) -> (133.934, -138.851)
  line L2390 (133.934, -138.851) -> (133.752, -139.068)
  line L2391 (131.271, -135.971) -> (131.522, -135.84)
  line L2392 (133.307, -139.413) -> (133.052, -139.535)
  line L2393 (134.312, -137.801) -> (134.274, -138.081)
  line L2394 (133.052, -139.535) -> (132.783, -139.621)
  line L2395 (132.783, -139.621) -> (132.504, -139.667)
  line L2396 (132.222, -139.674) -> (131.941, -139.64)
  line L2397 (133.837, -136.377) -> (134.005, -136.604)
  line L2398 (134.198, -138.353) -> (134.084, -138.612)
  line L2399 (130.947, -139.134) -> (130.755, -138.926)
  line L2400 (130.755, -138.926) -> (130.595, -138.694)
  line L2401 (201.788, -135.732) -> (202.07, -135.716)
  line L2402 (134.005, -136.604) -> (134.139, -136.853)
  line L2403 (200.101, -138.213) -> (200.051, -137.935)
  line L2404 (133.639, -136.176) -> (133.837, -136.377)
  line L2405 (200.051, -137.935) -> (200.039, -137.653)
  line L2406 (133.168, -135.866) -> (133.414, -136.004)
  line L2407 (200.478, -138.966) -> (200.317, -138.734)
  line L2408 (200.191, -138.481) -> (200.101, -138.213)
  line L2409 (200.764, -136.175) -> (200.994, -136.011)
  line L2410 (200.994, -136.011) -> (201.244, -135.88)
  line L2411 (133.414, -136.004) -> (133.639, -136.176)
  line L2412 (201.391, -139.608) -> (201.131, -139.498)
  line L2413 (130.595, -138.694) -> (130.468, -138.441)
  line L2414 (200.136, -137.098) -> (200.242, -136.836)
  line L2415 (134.316, -137.676) -> (134.312, -137.801)
  line L2416 (134.296, -137.394) -> (134.316, -137.676)
  line L2417 (200.559, -136.37) -> (200.764, -136.175)
  line L2418 (130.468, -138.441) -> (130.379, -138.173)
  line L2419 (132.504, -139.667) -> (132.222, -139.674)
  line L2420 (130.328, -137.895) -> (130.317, -137.613)
  line L2421 (134.274, -138.081) -> (134.198, -138.353)
  line L2422 (132.629, -135.7) -> (132.904, -135.764)
  line L2423 (133.752, -139.068) -> (133.542, -139.256)
  line L2424 (200.242, -136.836) -> (200.384, -136.592)
  line L2425 (130.52, -136.796) -> (130.662, -136.552)
  line L2426 (131.166, -139.312) -> (130.947, -139.134)
  line L2427 (201.244, -135.88) -> (201.511, -135.787)
  line L2428 (130.317, -137.613) -> (130.346, -137.332)
  line L2429 (134.237, -137.118) -> (134.296, -137.394)
  line L2430 (201.131, -139.498) -> (200.888, -139.352)
  line L2431 (130.379, -138.173) -> (130.328, -137.895)
  line L2432 (134.139, -136.853) -> (134.237, -137.118)
  line L2433 (130.662, -136.552) -> (130.837, -136.33)
  line L2434 (133.542, -139.256) -> (133.307, -139.413)
  line L2435 (131.941, -139.64) -> (131.668, -139.568)
  line L2436 (131.041, -136.135) -> (131.271, -135.971)
  line L2437 (131.668, -139.568) -> (131.408, -139.458)
  line L2438 (130.346, -137.332) -> (130.414, -137.058)
  line L2439 (131.408, -139.458) -> (131.166, -139.312)
  line L2440 (196.086, -138.585) -> (196.106, -138.4)
  line L2441 (197.71, -137.929) -> (197.827, -138.072)
  line L2442 (196.655, -139.469) -> (196.493, -139.378)
  line L2443 (196.352, -139.258) -> (196.237, -139.113)
  line L2444 (197.827, -138.072) -> (197.914, -138.236)
  line L2445 (196.101, -138.77) -> (196.086, -138.585)
  line L2446 (132.347, -135.676) -> (132.629, -135.7)
  line L2447 (197.016, -139.548) -> (196.832, -139.526)
  line L2448 (197.986, -138.598) -> (197.985, -138.625)
  line L2449 (197.379, -139.484) -> (197.201, -139.534)
  line L2450 (197.227, -137.667) -> (197.404, -137.722)
  line L2451 (196.493, -139.378) -> (196.352, -139.258)
  line L2452 (196.237, -139.113) -> (196.152, -138.948)
  line L2453 (136.436, -138.908) -> (136.384, -138.729)
  line L2454 (197.567, -137.81) -> (197.71, -137.929)
  line L2455 (197.812, -139.146) -> (197.691, -139.286)
  line L2456 (132.065, -135.692) -> (132.347, -135.676)
  line L2457 (197.404, -137.722) -> (197.567, -137.81)
  line L2458 (197.985, -138.625) -> (197.962, -138.808)
  line L2459 (137.974, -139.246) -> (137.828, -139.36)
  line L2460 (136.635, -139.218) -> (136.52, -139.073)
  line L2461 (196.162, -138.224) -> (196.252, -138.061)
  line L2462 (136.446, -138.184) -> (136.535, -138.021)
  line L2463 (196.832, -139.526) -> (196.655, -139.469)
  line L2464 (197.962, -138.808) -> (197.904, -138.984)
  line L2465 (131.788, -135.747) -> (132.065, -135.692)
  line L2466 (197.691, -139.286) -> (197.545, -139.4)
  line L2467 (138.251, -138.373) -> (138.269, -138.558)
  line L2468 (197.545, -139.4) -> (197.379, -139.484)
  line L2469 (197.904, -138.984) -> (197.812, -139.146)
  line L2470 (197.042, -137.648) -> (197.227, -137.667)
  line L2471 (137.687, -137.682) -> (137.85, -137.77)
  line L2472 (197.201, -139.534) -> (197.016, -139.548)
  line L2473 (197.914, -138.236) -> (197.968, -138.413)
  line L2474 (196.106, -138.4) -> (196.162, -138.224)
  line L2475 (131.522, -135.84) -> (131.788, -135.747)
  line L2476 (196.152, -138.948) -> (196.101, -138.77)
  line L2477 (196.252, -138.061) -> (196.371, -137.919)
  line L2478 (197.968, -138.413) -> (197.986, -138.598)
  line L2479 (138.269, -138.558) -> (138.268, -138.584)
  line L2480 (137.828, -139.36) -> (137.662, -139.444)
  line L2481 (136.938, -139.428) -> (136.777, -139.338)
  line L2482 (196.371, -137.919) -> (196.515, -137.803)
  line L2483 (137.115, -139.486) -> (136.938, -139.428)
  line L2484 (136.384, -138.729) -> (136.369, -138.545)
  line L2485 (136.369, -138.545) -> (136.39, -138.36)
  line L2486 (137.662, -139.444) -> (137.484, -139.494)
  line L2487 (317.904, -139.127) -> (317.623, -139.093)
  line L2488 (137.993, -137.889) -> (138.11, -138.032)
  line L2489 (138.245, -138.768) -> (138.187, -138.944)
  line L2490 (196.68, -137.717) -> (196.858, -137.665)
  line L2491 (138.268, -138.584) -> (138.245, -138.768)
  line L2492 (137.325, -137.608) -> (137.51, -137.627)
  line L2493 (319.998, -137.129) -> (319.994, -137.254)
  line L2494 (137.299, -139.508) -> (137.115, -139.486)
  line L2495 (136.39, -138.36) -> (136.446, -138.184)
  line L2496 (319.519, -135.83) -> (319.687, -136.057)
  line L2497 (318.465, -139.074) -> (318.186, -139.12)
  line L2498 (319.821, -136.306) -> (319.919, -136.571)
  line L2499 (196.858, -137.665) -> (197.042, -137.648)
  line L2500 (138.11, -138.032) -> (138.197, -138.196)
  line L2501 (319.321, -135.629) -> (319.519, -135.83)
  line L2502 (319.957, -137.534) -> (319.88, -137.806)
  line L2503 (137.85, -137.77) -> (137.993, -137.889)
  line L2504 (319.096, -135.457) -> (319.321, -135.629)
  line L2505 (319.994, -137.254) -> (319.957, -137.534)
  line L2506 (138.197, -138.196) -> (138.251, -138.373)
  line L2507 (318.85, -135.319) -> (319.096, -135.457)
  line L2508 (138.095, -139.106) -> (137.974, -139.246)
  line L2509 (137.141, -137.625) -> (137.325, -137.608)
  line L2510 (136.963, -137.677) -> (137.141, -137.625)
  line L2511 (317.35, -139.021) -> (317.09, -138.911)
  line L2512 (317.09, -138.911) -> (316.848, -138.765)
  line L2513 (319.978, -136.847) -> (319.998, -137.129)
  line L2514 (319.434, -138.521) -> (319.224, -138.709)
  line L2515 (318.186, -139.12) -> (317.904, -139.127)
  line L2516 (319.919, -136.571) -> (319.978, -136.847)
  line L2517 (137.484, -139.494) -> (137.299, -139.508)
  line L2518 (319.224, -138.709) -> (318.989, -138.866)
  line L2519 (319.88, -137.806) -> (319.766, -138.065)
  line L2520 (196.515, -137.803) -> (196.68, -137.717)
  line L2521 (136.777, -139.338) -> (136.635, -139.218)
  line L2522 (137.51, -137.627) -> (137.687, -137.682)
  line L2523 (136.52, -139.073) -> (136.436, -138.908)
  line L2524 (138.187, -138.944) -> (138.095, -139.106)
  line L2525 (316.15, -137.894) -> (316.061, -137.626)
  line L2526 (316.629, -138.587) -> (316.437, -138.379)
  line L2527 (16.9444, -135.177) -> (17.2078, -135.279)
  line L2528 (317.623, -139.093) -> (317.35, -139.021)
  line L2529 (317.748, -135.145) -> (318.03, -135.129)
  line L2530 (317.47, -135.2) -> (317.748, -135.145)
  line L2531 (17.4543, -135.417) -> (17.6789, -135.588)
  line L2532 (136.799, -137.763) -> (136.963, -137.677)
  line L2533 (319.687, -136.057) -> (319.821, -136.306)
  line L2534 (318.311, -135.153) -> (318.586, -135.217)
  line L2535 (318.989, -138.866) -> (318.734, -138.988)
  line L2536 (316.437, -138.379) -> (316.277, -138.147)
  line L2537 (317.204, -135.293) -> (317.47, -135.2)
  line L2538 (319.766, -138.065) -> (319.616, -138.304)
  line L2539 (16.6691, -135.113) -> (16.9444, -135.177)
  line L2540 (316.061, -137.626) -> (316.01, -137.348)
  line L2541 (18.1791, -136.266) -> (18.2769, -136.531)
  line L2542 (136.654, -137.879) -> (136.799, -137.763)
  line L2543 (136.535, -138.021) -> (136.654, -137.879)
  line L2544 (318.586, -135.217) -> (318.85, -135.319)
  line L2545 (318.734, -138.988) -> (318.465, -139.074)
  line L2546 (319.616, -138.304) -> (319.434, -138.521)
  line L2547 (316.723, -135.588) -> (316.953, -135.423)
  line L2548 (316.028, -136.785) -> (316.096, -136.511)
  line L2549 (315.999, -137.066) -> (316.028, -136.785)
  line L2550 (316.848, -138.765) -> (316.629, -138.587)
  line L2551 (14.5085, -137.854) -> (14.4191, -137.586)
  line L2552 (17.8771, -135.79) -> (18.0449, -136.017)
  line L2553 (18.238, -137.766) -> (18.1238, -138.025)
  line L2554 (16.8232, -139.033) -> (16.5445, -139.08)
  line L2555 (14.3683, -137.308) -> (14.3573, -137.026)
  line L2556 (15.0814, -135.548) -> (15.3113, -135.383)
  line L2557 (316.344, -136.005) -> (316.519, -135.783)
  line L2558 (18.0449, -136.017) -> (18.1791, -136.266)
  line L2559 (14.7954, -138.339) -> (14.6348, -138.107)
  line L2560 (15.4483, -138.871) -> (15.2063, -138.725)
  line L2561 (316.953, -135.423) -> (317.204, -135.293)